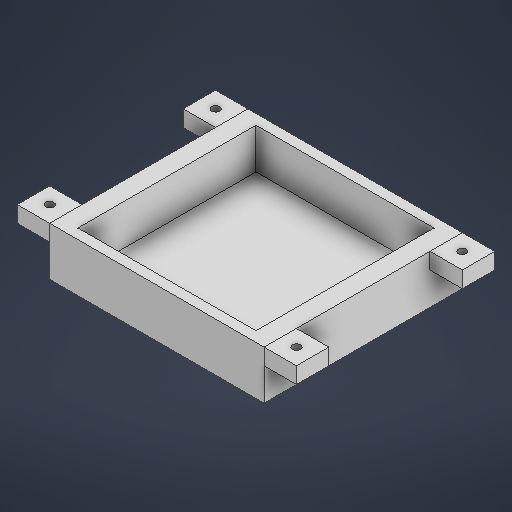
# Autodesk Inventor part: Oberteil
Saved by Autodesk Inventor 2026.2 (Build 302298000, 298)
## iProperties
Created: 2026-04-09
Part Number: Oberteil
Material: Generisch
Document SubType Name: Modeling
Designer: linda
Density: 1 g/cm^3
Appearance: Vorgabe
Author: linda
Autodesk Inventor part; units mm, degrees
ref_plane "YZ Plane" through (0, 0, 0) normal (1, 0, 0) x (0, 1, 0)
ref_plane "XZ Plane" through (0, 0, 0) normal (0, 1, 0) x (-1, 0, 0)
ref_plane "XY Plane" through (0, 0, 0) normal (0, 0, 1) x (1, 0, 0)
sketch "Skizze1" plane through (0, 0, 0) normal (0, 1, 0) x (-1, 0, 0)
  line L0 (0, 0) -> (-132.5, 0)
  line L1 (-132.5, 0) -> (-132.5, 122.5)
  line L2 (-132.5, 122.5) -> (0, 122.5)
  line L3 (0, 122.5) -> (0, 0)
  dimension "d0" = 132.5
  dimension "d1" = 122.5
  constraints: 8 end point, 2 parallel, 1 horizontal, 1 perpendicular
  measures "d0" distance of L1.end L2.end
  measures "d1" distance of L0.end L1.end
extrude "Extrusion1" add sketch "Skizze1" along normal blind 30
sketch "Skizze2" plane through (0, 30, 0) normal (0, 1, 0) x (1, 0, 0)
  line L0 (0, 0) -> (11.25, 0)
  line L1 (11.25, 0) -> (11.25, -6.25)
  line L2 (11.25, -6.25) -> (121.25, -6.25)
  line L3 (121.25, -6.25) -> (121.25, -116.25)
  line L4 (121.25, -116.25) -> (11.25, -116.25)
  line L5 (11.25, -116.25) -> (11.25, -6.25)
  dimension "d4" = 11.25
  dimension "d5" = 6.25
  dimension "d6" = 110
  dimension "d7" = 110
  constraints: 12 end point, 2 horizontal, 2 parallel, 2 perpendicular
  measures "d4" distance of L0.start L0.end
  measures "d5" distance of L0.end L1.end
  measures "d6" distance of L3.end L4.end
  measures "d7" distance of L2.end L3.end
extrude "Extrusion2" cut sketch "Skizze2" against normal blind 25
sketch "Skizze3" plane through (0, 0, 0) normal (-1, 0, 0) x (0, 0, 1)
  line L0 (0, 29.9998) -> (20, 29.9998)
  line L1 (20, 29.9998) -> (20, 19.9998)
  line L2 (20, 19.9998) -> (0, 19.9998)
  line L3 (0, 19.9998) -> (0, 29.9998)
  line L4 (122.5002, 29.9998) -> (102.5002, 29.9998)
  line L5 (102.5002, 29.9998) -> (102.5002, 19.9998)
  line L6 (102.5002, 19.9998) -> (122.5002, 19.9998)
  line L7 (122.5002, 19.9998) -> (122.5002, 29.9998)
  point P0 (0, 0)
  dimension "d10" = 20
  dimension "d11" = 10
  dimension "d12" = 20
  dimension "d13" = 10
  constraints: 16 end point, 4 parallel, 2 horizontal, 2 perpendicular, 1 point on line
  measures "d10" distance of L1.end L2.end
  measures "d11" distance of L0.end L1.end
  measures "d12" distance of L6.end L5.end
  measures "d13" distance of L5.end L4.end
extrude "Extrusion3" add sketch "Skizze3" along normal blind 20
sketch "Skizze4" plane through (132.5, 0, 122.5) normal (1, 0, 0) x (0, 0, -1)
  line L0 (0.0001, 29.9997) -> (20.0001, 29.9997)
  line L1 (20.0001, 29.9997) -> (20.0001, 19.9997)
  line L2 (20.0001, 19.9997) -> (0.0001, 19.9997)
  line L3 (0.0001, 19.9997) -> (0.0001, 29.9997)
  line L4 (122.5, 29.9997) -> (102.5, 29.9997)
  line L5 (102.5, 29.9997) -> (102.5, 19.9997)
  line L6 (102.5, 19.9997) -> (122.5, 19.9997)
  line L7 (122.5, 19.9997) -> (122.5, 29.9997)
  point P0 (122.5, 0)
  dimension "d16" = 20
  dimension "d17" = 10
  dimension "d18" = 20
  dimension "d19" = 10
  constraints: 16 end point, 4 parallel, 2 horizontal, 2 perpendicular, 1 point on line
  measures "d16" distance of L1.end L2.end
  measures "d17" distance of L0.end L1.end
  measures "d18" distance of L6.end L5.end
  measures "d19" distance of L5.end L4.end
extrude "Extrusion4" add sketch "Skizze4" along normal blind 20
sketch "Skizze5" plane through (0, 29.9998, 122.5) normal (0, 1, 0) x (1, 0, 0)
  line L0 (0, 19.9998) -> (-20, 19.9998) projected
  line L1 (-20, -0.0002) -> (-20, 19.9998) projected
  point P0 (0, 122.5)
  point P1 (-10, 9.9998)
  dimension "d22" = 10
  dimension "d23" = 10
  measures "d22" distance from line of L0 point (-10, 10)
  measures "d23" distance from line of L1 point (-10, 10)
hole "Bohrung1" at (-10, 29.9998, 112.5002) direction (0, -1, 0) diameter 5 end through all
sketch "Skizze6" plane through (0, 29.9998, 20) normal (0, 1, 0) x (1, 0, 0)
  line L0 (0, 20) -> (-20, 20) projected
  line L1 (-20, 0) -> (-20, 20) projected
  point P0 (-10, 10)
  dimension "d31" = 10
  dimension "d32" = 10
  measures "d31" distance from line of L0 point (-10, 10)
  measures "d32" distance from line of L1 point (-10, 10)
hole "Bohrung2" at (-10, 29.9998, 10) direction (0, -1, 0) diameter 5 end through all
sketch "Skizze7" plane through (132.5, 29.9997, 122.4999) normal (0, 1, 0) x (1, 0, 0)
  line L0 (0, 20) -> (20, 20) projected
  line L1 (20, 20) -> (20, 0) projected
  point P0 (-132.5, 122.4999)
  point P1 (10, 10)
  dimension "d40" = 10
  dimension "d41" = 10
  measures "d40" distance from line of L0 point (10, 10)
  measures "d41" distance from line of L1 point (10, 10)
hole "Bohrung3" at (142.5, 29.9997, 112.4999) direction (0, -1, 0) diameter 5 end through all
sketch "Skizze8" plane through (132.5, 29.9997, 20) normal (0, 1, 0) x (1, 0, 0)
  line L0 (0, 20) -> (20, 20) projected
  line L1 (20, 20) -> (20, 0) projected
  point P0 (-132.5, 20)
  point P1 (10, 10)
  dimension "d49" = 10
  dimension "d50" = 10
  measures "d49" distance from line of L0 point (10, 10)
  measures "d50" distance from line of L1 point (10, 10)
hole "Bohrung4" at (142.5, 29.9997, 10) direction (0, -1, 0) diameter 5 end through all
thread "Gewinde1" size "M5x0.8" class "6H" standard "ANSI Metric M Profile" full length
thread "Gewinde2" size "M5x0.8" class "6H" standard "ANSI Metric M Profile" full length
thread "Gewinde3" size "M5x0.8" class "6H" standard "ANSI Metric M Profile" full length
thread "Gewinde4" size "M5x0.8" class "6H" standard "ANSI Metric M Profile" full length
